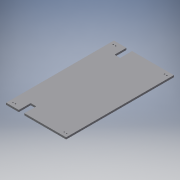
# Autodesk Inventor part: étage
Saved by Autodesk Inventor 2019 (Build 230136000, 136)
## iProperties
Created: 2019-03-31
Part Number: étage
Material: Generic
Document SubType Name: Modeling
Designer: franc
Density: 1 g/cm^3
Appearance: Default
Author: franc
Autodesk Inventor part; units mm, degrees
ref_plane "YZ Plane" through (0, 0, 0) normal (1, 0, 0) x (0, 1, 0)
ref_plane "XZ Plane" through (0, 0, 0) normal (0, 1, 0) x (-1, 0, 0)
ref_plane "XY Plane" through (0, 0, 0) normal (0, 0, 1) x (1, 0, 0)
sketch "Esquisse1" plane through (0, 0, 0) normal (0, 1, 0) x (-1, 0, 0)
  line L0 (94.7405, 132.2434) -> (-66.7595, 132.2434)
  line L1 (-66.7595, 132.2434) -> (-66.7595, -157.7566)
  line L2 (-66.7595, -157.7566) -> (94.7405, -157.7566)
  line L3 (94.7405, -157.7566) -> (94.7405, 132.2434)
  point P0 (0, 0)
  dimension "d0" = 290
  dimension "d1" = 161.5
  constraints: 8 end point, 2 parallel, 1 horizontal, 1 perpendicular
  measures "d0" distance of L0.end L1.end
  measures "d1" distance of L1.end L2.end
extrude "Extrusion1" add sketch "Esquisse1" along normal blind 5
sketch "Esquisse3" plane through (0, 5, 0) normal (0, 1, 0) x (1, 0, 0)
  circle A0 centre (58.2595, 147.7566) radius 1.5 projected
  circle A1 centre (51.7595, 147.7566) radius 1.5 projected
  circle A2 centre (58.2595, -122.2434) radius 1.5 projected
  circle A3 centre (51.7595, -122.2434) radius 1.5 projected
  line L0 (-13.9905, 179.8328) -> (-13.9905, -180.1419)
  line L1 (66.7595, -132.2434) -> (66.7595, 157.7566) projected
  circle A4 centre (-86.2405, 147.7566) radius 1.5
  circle A5 centre (-79.7405, 147.7566) radius 1.5
  circle A6 centre (-86.2405, -122.2434) radius 1.5
  circle A7 centre (-79.7405, -122.2434) radius 1.5
  point P0 (0, 0)
  dimension "d11" = 80.75
  constraints: 4 centre point, 4 symmetric about line, 2 end point, 1 vertical, 4 other
  measures "d11" distance between parallel lines of L1 L0
extrude "Extrusion3" cut sketch "Esquisse3" against normal up to next
sketch "Esquisse4" plane through (0, 5, 0) normal (0, 1, 0) x (1, 0, 0)
  line L0 (-94.7405, -132.2434) -> (66.7595, -132.2434) projected
  line L1 (-60.7405, -100.2434) -> (-45.7405, -100.2434)
  line L2 (-45.7405, -100.2434) -> (-45.7405, -132.2434)
  line L3 (-45.7405, -132.2434) -> (-60.7405, -132.2434)
  line L4 (-60.7405, -132.2434) -> (-60.7405, -100.2434)
  line L5 (-94.7405, 157.7566) -> (-94.7405, -132.2434) projected
  line L6 (-60.7405, 125.7566) -> (-45.7405, 125.7566)
  line L7 (-45.7405, 125.7566) -> (-45.7405, 157.7566)
  line L8 (-45.7405, 157.7566) -> (-60.7405, 157.7566)
  line L9 (-60.7405, 157.7566) -> (-60.7405, 125.7566)
  line L10 (66.7595, 157.7566) -> (-94.7405, 157.7566) projected
  point P0 (0, 0)
  dimension "d12" = 15
  dimension "d13" = 32
  dimension "d14" = 34
  dimension "d15" = 34
  dimension "d16" = 15
  dimension "d17" = 32
  dimension "d18" = 0
  constraints: 16 end point, 4 parallel, 2 horizontal, 2 perpendicular, 1 point on line
  measures "d12" distance of L1.start L1.end
  measures "d13" distance of L3.end L1.start
  measures "d14" distance between parallel lines of L5 L4
  measures "d15" distance between parallel lines of L5 L9
  measures "d16" distance of L6.start L6.end
  measures "d17" distance of L8.end L6.start
  measures "d18" distance between parallel lines of L10 L8
extrude "Extrusion4" cut sketch "Esquisse4" against normal through all
